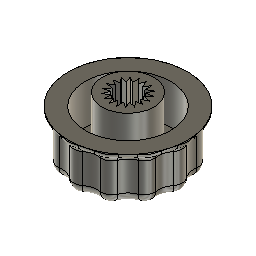
front2_dev (Autodesk Fusion 360 archive; units mm, degrees)
design "volume_knob"
Autodesk Fusion 360 part; units mm, degrees
sketch "Skizze1" plane through (0, 0, 0) normal (0, 0, 1) x (1, 0, 0)
  arc A0 (3.951698, -9.338845) -> (2.523801, -9.418955) centre (3.429668, -12.799695) ccw
  circle A1 centre (0, 0) radius 5
  line L0 (-1.356886, -7.695284) -> (1.126342, 6.387801) construction
  line L1 (5.775232, 21.553458) -> (-3.705632, -13.829606) construction
  arc A2 (6.895153, -6.895153) -> (6.111828, -8.091692) centre (9.370027, -9.370027) ccw
  line L2 (2.4, -0.000006) -> (3.545308, -0.625133)
  arc A3 (-1.247152, -10.063526) -> (1.247152, -10.063525) centre (0, -8.5) ccw
  arc A4 (-9.418955, -2.523801) -> (-10.063525, -1.247152) centre (-12.799695, -3.429668) ccw
  line L3 (2.25526, -0.820854) -> (3.117691, -1.8)
  line L4 (-0.416762, -2.363537) -> (-1.231273, -3.382893)
  line L5 (-5.895645, 22.002848) -> (3.63479, -13.565219) construction
  line L6 (3.117691, -1.8) -> (1.838507, -1.54269)
  arc A5 (10.063526, -1.247152) -> (10.063525, 1.247152) centre (8.5, 0) ccw
  circle A6 centre (0, 0) radius 2.4 construction
  circle A7 centre (0, 0) radius 11.5
  circle A8 centre (0, 0) radius 10.5 construction
  line L7 (0, -60.68219) -> (0, 59.394716) construction
  circle A9 centre (0, 0) radius 8.25
  line L8 (-3.545308, -0.625133) -> (-2.4, 0)
  line L9 (-1.83851, -1.542686) -> (-3.117691, -1.8)
  circle A10 centre (0, 0) radius 3.6 construction
  line L10 (-2.255264, -0.820843) -> (-3.545308, -0.625133)
  arc A11 (-10.063526, 1.247152) -> (-10.063525, -1.247152) centre (-8.5, 0) ccw
  arc A12 (3.951698, -9.338845) -> (6.111828, -8.091692) centre (4.25, -7.361216) ccw
  line L11 (-1.165017, 6.60714) -> (1.472183, -8.349163) construction
  arc A13 (-2.523801, -9.418955) -> (-3.951697, -9.338845) centre (-3.429668, -12.799695) ccw
  line L12 (3.545308, -0.625133) -> (2.255262, -0.820848)
  line L13 (1.838503, -1.542695) -> (2.314035, -2.75776)
  line L14 (0, -3.6) -> (-0.416756, -2.363539)
  line L15 (0.41675, -2.36354) -> (0, -3.6)
  arc A14 (-6.111828, -8.091693) -> (-3.951697, -9.338845) centre (-4.25, -7.361216) ccw
  arc A15 (-9.338845, -3.951698) -> (-8.091692, -6.111828) centre (-7.361216, -4.25) ccw
  line L16 (-1.231273, -3.382893) -> (-1.2, -2.078461)
  line L17 (-3.117691, -1.8) -> (-2.255262, -0.820848)
  arc A16 (2.523801, -9.418955) -> (1.247152, -10.063525) centre (3.429668, -12.799695) ccw
  line L18 (2.314035, -2.75776) -> (1.2, -2.078461)
  arc A17 (8.091693, -6.111828) -> (9.338845, -3.951697) centre (7.361216, -4.25) ccw
  arc A18 (-9.338845, -3.951698) -> (-9.418955, -2.523801) centre (-12.799695, -3.429668) ccw
  line L19 (-1.200005, -2.078458) -> (-2.314035, -2.75776)
  arc A19 (-8.091693, 6.111828) -> (-9.338845, 3.951697) centre (-7.361216, 4.25) ccw
  line L20 (-2.314035, -2.75776) -> (-1.838507, -1.54269)
  arc A20 (9.338845, 3.951698) -> (8.091692, 6.111828) centre (7.361216, 4.25) ccw
  arc A21 (-1.247152, -10.063526) -> (-2.523801, -9.418955) centre (-3.429668, -12.799695) ccw
  arc A22 (-10.063526, 1.247152) -> (-9.418955, 2.523801) centre (-12.799695, 3.429668) ccw
  arc A23 (-6.895153, -6.895153) -> (-8.091692, -6.111828) centre (-9.370027, -9.370027) ccw
  line L21 (-0.41675, 2.36354) -> (0, 3.6)
  circle A24 centre (0, 8.5) radius 2 construction
  arc A25 (10.063526, -1.247152) -> (9.418955, -2.523801) centre (12.799695, -3.429668) ccw
  line L22 (-1.838503, 1.542695) -> (-2.314035, 2.75776)
  arc A26 (-8.091693, 6.111828) -> (-6.895153, 6.895153) centre (-9.370027, 9.370027) ccw
  arc A27 (8.091693, -6.111828) -> (6.895153, -6.895153) centre (9.370027, -9.370027) ccw
  arc A28 (-6.895153, 6.895153) -> (-6.111828, 8.091692) centre (-9.370027, 9.370027) ccw
  line L23 (1.231273, -3.382893) -> (0.416756, -2.363539)
  arc A29 (1.247152, 10.063526) -> (2.523801, 9.418955) centre (3.429668, 12.799695) ccw
  arc A30 (9.418955, 2.523801) -> (10.063525, 1.247152) centre (12.799695, 3.429668) ccw
  arc A31 (-6.111828, -8.091693) -> (-6.895153, -6.895153) centre (-9.370027, -9.370027) ccw
  line L24 (-1.231273, 3.382893) -> (-0.416756, 2.363539)
  arc A32 (6.111828, 8.091693) -> (3.951697, 9.338845) centre (4.25, 7.361216) ccw
  arc A33 (9.418955, -2.523801) -> (9.338845, -3.951697) centre (12.799695, -3.429668) ccw
  circle A34 centre (3.429668, 12.799695) radius 3.5 construction
  line L25 (1.199995, -2.078464) -> (1.231273, -3.382893)
  arc A35 (-3.951698, 9.338845) -> (-2.523801, 9.418955) centre (-3.429668, 12.799695) ccw
  arc A36 (1.247152, 10.063526) -> (-1.247152, 10.063525) centre (0, 8.5) ccw
  line L26 (2.255264, 0.820843) -> (3.545308, 0.625133)
  line L27 (-2.314035, 2.75776) -> (-1.2, 2.078461)
  circle A37 centre (-3.429668, 12.799695) radius 3.5 construction
  arc A38 (6.895153, 6.895153) -> (8.091692, 6.111828) centre (9.370027, 9.370027) ccw
  arc A39 (2.523801, 9.418955) -> (3.951697, 9.338845) centre (3.429668, 12.799695) ccw
  arc A40 (6.111828, 8.091693) -> (6.895153, 6.895153) centre (9.370027, 9.370027) ccw
  line L28 (-2.25526, 0.820854) -> (-3.117691, 1.8)
  arc A41 (-9.418955, 2.523801) -> (-9.338845, 3.951697) centre (-12.799695, 3.429668) ccw
  arc A42 (-2.523801, 9.418955) -> (-1.247152, 10.063525) centre (-3.429668, 12.799695) ccw
  arc A43 (-3.951698, 9.338845) -> (-6.111828, 8.091692) centre (-4.25, 7.361216) ccw
  line L29 (1.200005, 2.078458) -> (2.314035, 2.75776)
  arc A44 (9.338845, 3.951698) -> (9.418955, 2.523801) centre (12.799695, 3.429668) ccw
  line L30 (0.416762, 2.363537) -> (1.231273, 3.382893)
  line L31 (2.314035, 2.75776) -> (1.838507, 1.54269)
  line L32 (1.231273, 3.382893) -> (1.2, 2.078461)
  line L33 (3.117691, 1.8) -> (2.255262, 0.820848)
  line L34 (0, 3.6) -> (0.416756, 2.363539)
  line L35 (-2.4, 0.000006) -> (-3.545308, 0.625133)
  line L36 (1.83851, 1.542686) -> (3.117691, 1.8)
  line L37 (-3.545308, 0.625133) -> (-2.255262, 0.820848)
  line L38 (-1.199995, 2.078464) -> (-1.231273, 3.382893)
  line L39 (-3.117691, 1.8) -> (-1.838507, 1.54269)
  line L40 (3.545308, 0.625133) -> (2.4, 0)
  line L41 (-196.099114, 0) -> (114.973446, 0) construction
  point P0 (-1.247152, 10.063525)
  point P1 (1.247152, 10.063526)
  dimension "d2" = 360
  dimension "d4" = 360
  dimension "d5" = 7.2
  dimension "d6" = 1.2
  dimension "d7" = 10
  dimension "d8" = 10
  dimension "d9" = 10
  dimension "d10" = 16.5
  dimension "d11" = 21
  dimension "d12" = 23
  dimension "d13" = 4
  dimension "d14" = 15
  dimension "d15" = 7
  dimension "d16" = 15
  dimension "d17" = 7
  constraint horizontal L41
  constraint vertical L7
  constraint coincident A1.centre L41
  constraint coincident A1.centre L7
  constraint concentric A6 A10
  constraint coincident A1.centre L11
  constraint coincident A1.centre L0
  constraint coincident L21.end A10
  constraint coincident L21.end L7
  constraint concentric A1 A10
  constraint concentric A9 A10
  constraint concentric A1 A8
  constraint concentric A6 A7
  constraint coincident A24.centre L7
  constraint tangent A8 A24
  constraint coincident A1.centre L1
  constraint tangent A24 A34
  constraint coincident A1.centre L5
  constraint tangent A24 A37
  constraint coincident A24.centre A36.centre
  measures "d5" diameter of A10
  measures "d6" distance of A6 A10
  measures "d7" angle of L7 L11
  measures "d8" angle of L0 L7
  measures "d9" diameter of A1
  measures "d10" diameter of A9
  measures "d11" diameter of A8
  measures "d12" diameter of A7
  measures "d13" diameter of A24
  measures "d14" angle of L1 L7
  measures "d15" diameter of A34
  measures "d16" angle of L5 L7
  measures "d17" diameter of A37
extrude "Extrusion1" add sketch "Skizze1" along normal blind 10 contours A1 picked at (-2.015103, -3.49026)
extrude "Extrusion2" add sketch "Skizze1" against normal blind 2 contours A0 A2 A3 A4 A5 A11 A12 A13 A14 A15 A16 A17 A18 A19 A20 A21 A22 A23 A25 A26 A27 A28 A29 A30 A31 A32 A33 A35 A36 A38 A39 A40 A41 A42 A43 A44 | A1 | L2 L3 L4 L6 L8 L9 L10 L12 L13 L14 L15 L16 L17 L18 L19 L20 L21 L22 L23 L24 L25 L26 L27 L28 L29 L30 L31 L32 L33 L34 L35 L36 L37 L38 L39 L40 | A9 picked at (-7.804209, -4.448226) picked at (-2.015103, -3.49026) picked at (-0.612834, 0.514232) picked at (7.135951, -0.409866)
extrude "Extrusion3" add sketch "Skizze1" along normal blind 7.7 contours A0 A2 A3 A4 A5 A11 A12 A13 A14 A15 A16 A17 A18 A19 A20 A21 A22 A23 A25 A26 A27 A28 A29 A30 A31 A32 A33 A35 A36 A38 A39 A40 A41 A42 A43 A44 | A7 picked at (-7.804209, -4.448226) picked at (10.645073, 2.391233)
extrude "Extrusion4" cut sketch "Skizze1" along normal blind 6.7 contours A7 picked at (10.645073, 2.391233)
fillet "Abrundung1" radius 1 1 faces at (10.645073, 2.391233, 6.7)
fillet "Abrundung2" radius 2 1 faces at (-0.61585, 2.298384, -2)

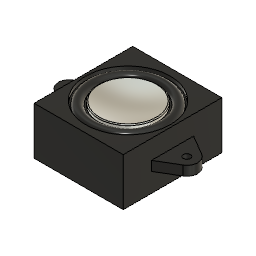
design "speaker_large"
Autodesk Fusion 360 part; units mm, degrees
sketch "Skizze1" plane through (0, 0, 0) normal (0, 0, 1) x (1, 0, 0)
  line L0 (0, 62.2181) -> (0, -52.8791) construction
  line L1 (-55.5293, 0) -> (56.0341, 0) construction
  line L2 (-14, 15.5) -> (-14, -15.5)
  line L3 (14, 15.5) -> (14, -15.5)
  line L4 (-14, 15.5) -> (14, 15.5)
  line L5 (-14, -15.5) -> (14, -15.5)
  circle A0 centre (18.5, 0) radius 1.1
  circle A1 centre (-18.5, 0) radius 1.1
  line L6 (21.9, 8) -> (21.9, -8) construction
  line L7 (-21.9, 8.3414) -> (-21.9, -9.3586) construction
  line L8 (-25.5548, 6.6) -> (28, 6.6) construction
  line L9 (-25.9053, -6.6) -> (28, -6.6) construction
  circle A2 centre (18.5, 0) radius 3.4 construction
  circle A3 centre (-18.5, 0) radius 3.4 construction
  line L10 (14, -6.6) -> (20.2268, -2.9289)
  line L11 (14, 6.6) -> (20.2268, 2.9289)
  line L12 (-14, 6.6) -> (-20.2268, 2.9289)
  line L13 (-14, -6.6) -> (-20.2268, -2.9289)
  arc A4 (-20.2268, 2.9289) -> (-20.2268, -2.9289) centre (-18.5, 0) ccw
  arc A5 (20.2268, -2.9289) -> (20.2268, 2.9289) centre (18.5, 0) ccw
  circle A6 centre (0, 0) radius 13.25
  circle A7 centre (18.5, 0) radius 4.4 construction
  line L14 (15, -7.1713) -> (20.7347, -3.7903) construction
  line L15 (15, -7.1713) -> (15, -16.5) construction
  line L16 (-9.5592, -16.5) -> (15, -16.5) construction
  point P0 (18.5, 0)
  point P1 (-18.5, 0)
  dimension "d1" = 14
  dimension "d2" = 14
  dimension "d3" = 15.5
  dimension "d4" = 15.5
  dimension "d5" = 18.5
  dimension "d6" = 18.5
  dimension "d7" = 2.2
  dimension "d8" = 2.2
  dimension "d9" = 21.9
  dimension "d10" = 21.9
  dimension "d11" = 6.6
  dimension "d12" = 6.6
  dimension "d13" = 26.5
  dimension "d30" = 8.8
  dimension "d31" = 1
  dimension "d32" = 1
  dimension "d33" = 5.7347
  dimension "d34" = 16.5
  dimension "d36" = 2.8097
  dimension "d37" = 9.3287
  constraint vertical L0
  constraint horizontal L1
  constraint coincident A6.centre L1
  constraint coincident A6.centre L0
  constraint vertical L2
  constraint vertical L3
  constraint horizontal L4
  constraint perpendicular L3 L5
  constraint coincident L3.end L5.end
  constraint coincident L2.end L5.start
  constraint coincident L2.start L4.start
  constraint coincident L3.start L4.end
  constraint coincident L1 P0
  constraint coincident L1 P1
  constraint coincident P0 A0.centre
  constraint coincident P1 A1.centre
  constraint vertical L6
  constraint perpendicular L1 L7
  constraint perpendicular L6 L8
  constraint horizontal L9
  constraint concentric A0 A2
  constraint concentric A1 A3
  constraint tangent L6 A2
  constraint tangent L7 A3
  constraint coincident L9 L10.start
  constraint coincident L3 L10.start
  constraint coincident L8 L11.start
  constraint coincident L3 L11.start
  constraint coincident L2 L12.start
  constraint coincident L8 L12.start
  constraint coincident L2 L13.start
  constraint coincident L9 L13.start
  constraint tangent A3 L13
  constraint tangent A3 L12
  constraint tangent A2 L10
  constraint tangent A2 L11
  constraint coincident A2 L11.end
  constraint coincident A2 L10.end
  constraint coincident A3 L13.end
  constraint coincident A3 L12.end
  constraint coincident L10 A5.start
  constraint coincident L11 A5.end
  constraint coincident L12 A4.start
  constraint coincident L13 A4.end
  constraint coincident A6.centre origin
  constraint parallel L10 L14
  constraint tangent A7 L14
  constraint coincident A7 L14.end
  constraint parallel L3 L15
  constraint perpendicular L15 L16
  constraint coincident L15.end L16.end
  measures "d1" distance of L0 L2
  measures "d2" distance of L0 L3
  measures "d3" distance of L1 L4
  measures "d4" distance of L1 L5
  measures "d5" distance of A6.centre P1
  measures "d6" distance of A6.centre A0.centre
  measures "d7" diameter of A1
  measures "d8" diameter of A0
  measures "d9" distance of A6.centre L7
  measures "d10" distance of L0 L6
  measures "d11" distance of L1 L8
  measures "d12" distance of L1 L9
  measures "d13" diameter of A6
  measures "d30" diameter of A7
  measures "d31" distance of L3 L15
  measures "d32" distance of L5 L16
  measures "d33" distance of L14.end L15
  measures "d34" distance of A6.centre L16
  measures "d36" distance of L9 L14.end
  measures "d37" distance of L14.start L16
extrude "Extrusion1" add sketch "Skizze1" along normal mid plane 15 contours L2 L3 L4 L5 makes body 1
extrude "Extrusion2" add sketch "Skizze1" against normal blind 7.5 contours A6 bodies 1
extrude "Extrusion3" add sketch "Skizze1" along normal mid plane 3 contours L2 L12 L13 A4 | L3 L10 L11 A5 bodies 1
sketch "Skizze2" plane through (0, 0, 0) normal (0, 1, 0) x (1, 0, 0)
  line L0 (-22.6965, -7.5) -> (25.4478, -7.5) construction
  line L1 (13.25, -11.5139) -> (13.25, 4.4454) construction
  line L2 (-8, -6) -> (18.2277, -6) construction
  circle A0 centre (11.25, -6) radius 1.5
  line L3 (13.25, -5.75) -> (9.25, -5.75)
  line L4 (9.25, -5.75) -> (9.25, -6.25)
  line L5 (9.25, -6.25) -> (13.25, -6.25)
  line L6 (13.25, -6.25) -> (13.25, -5.75)
  line L7 (13.25, -5.75) -> (9.25, -6.25) construction
  line L8 (9.25, -5.75) -> (13.25, -6.25) construction
  line L9 (9.25, -5.75) -> (0, -5.75)
  line L10 (0, -5.75) -> (0, -7.5)
  line L11 (0, -7.5) -> (9.25, -7.5)
  line L12 (9.25, -7.5) -> (9.25, -5.75)
  line L13 (0, -30.6693) -> (0, 1.4469) construction
  arc A1 (9.25, -7.5) -> (0, -6.2093) centre (0, -40) ccw
  circle A2 centre (9, -7.1706) radius 0.25 construction
  arc A3 (8.9339, -7.4117) -> (9.25, -7.1706) centre (9, -7.1706) ccw
  point P0 (11.25, -6)
  dimension "d20" = 7.5
  dimension "d21" = 13.25
  dimension "d22" = 3
  dimension "d23" = 4
  dimension "d24" = 0.5
  dimension "d25" = 40
  dimension "d26" = 0.5
  constraint horizontal L0
  constraint vertical L1
  constraint horizontal L2
  constraint coincident L2 P0
  constraint tangent L0 A0
  constraint horizontal L3
  constraint perpendicular L3 L4
  constraint parallel L3 L5
  constraint parallel L4 L6
  constraint coincident L7 P0
  constraint coincident L8 P0
  constraint coincident P0 A0.centre
  constraint coincident L1 L3.start
  constraint horizontal L9
  constraint vertical L10
  constraint horizontal L11
  constraint vertical L12
  constraint coincident L0 L10.end
  constraint vertical L13
  constraint coincident origin L13
  constraint coincident L13 A1.end
  constraint coincident L13 A1.centre
  constraint tangent A1 A2
  constraint tangent L12 A2
  constraint coincident A2 A3.end
  constraint coincident A2 A3.start
  constraint coincident A2.centre A3.centre
  constraint coincident A1 A3.start
  constraint coincident L12 A3.end
  measures "d20" distance of origin L0
  measures "d21" distance of origin L1
  measures "d22" diameter of A0
  measures "d23" distance of L4 L6
  measures "d24" distance of L3 L5
  measures "d25" distance of origin A1.centre
  measures "d26" diameter of A2
revolve "Drehen2" add sketch "Skizze2" angle 360 about axis through (0, 0, 30.6693) along (0, 0, -1) contours A0 L3 L5 | A0 L3 L5 L6 | A0 L3 | A0 L5 | A0 L3 L4 L5 L12 bodies 1
revolve "Drehen3" add sketch "Skizze2" angle 360 about axis through (0, 0, 30.6693) along (0, 0, -1) separate body contours L4 L9 L10 L12 A1 A3 makes body 2
equation "d5 = ( 37 / 2 ) * 1 mm"
equation "d6 = ( 37 / 2 ) * 1 mm"
equation "d9 = ( 43.8 / 2 ) * 1 mm"
equation "d10 = ( 43.8 / 2 ) * 1 mm"
equation "d11 = ( 13.2 / 2 ) * 1 mm"
equation "d12 = ( 13.2 / 2 ) * 1 mm"
equation "d21 = ( 26.5 / 2 ) * 1 mm"
named bodies: "case", "membrane"
